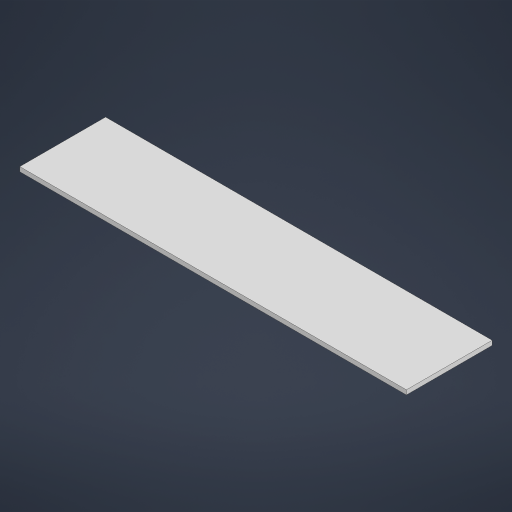
# Autodesk Inventor part: platte2
Saved by Autodesk Inventor 2023 (Build 270158000, 158)
## iProperties
Created: 2022-09-26
Part Number: platte2
Material: Generic
Document SubType Name: Modeling
Designer: bananenbrot
Density: 1 g/cm^3
Appearance: Default
Author: bananenbrot
Autodesk Inventor part; units mm, degrees
ref_plane "YZ Plane" through (0, 0, 0) normal (1, 0, 0) x (0, 1, 0)
ref_plane "XZ Plane" through (0, 0, 0) normal (0, 1, 0) x (-1, 0, 0)
ref_plane "XY Plane" through (0, 0, 0) normal (0, 0, 1) x (1, 0, 0)
sketch "Sketch1" plane through (0, 0, 0) normal (1, 0, 0) x (0, 1, 0)
  line L0 (11.0334, 50.0976) -> (7.7334, 50.0976)
  line L1 (7.7334, 50.0976) -> (7.7334, -13.8024)
  line L2 (7.7334, -13.8024) -> (11.0334, -13.8024)
  line L3 (11.0334, -13.8024) -> (11.0334, 50.0976)
  point P0 (0, 0)
  dimension "d0" = 63.9
  dimension "d1" = 3.3
  constraints: 8 end point, 2 parallel, 1 horizontal, 1 perpendicular
  measures "d0" distance of L2.end L0.start
  measures "d1" distance of L1.end L2.end
extrude "Extrusion1" add sketch "Sketch1" along normal blind 288
body "Solid1"
